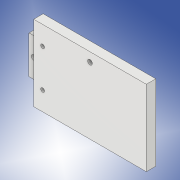
# Autodesk Inventor part: SP001
Saved by Autodesk Inventor 2017 SP1 (Build 210196100, 196)
## iProperties
Created: 2017-08-09
Part Number: SP001
Material: ABS Plastic
Document SubType Name: Modeling
Designer: Zach
Density: 1.06 g/cm^3
Appearance: CR White
Author: Zach
Autodesk Inventor part; units mm, degrees
ref_plane "YZ Plane" through (0, 0, 0) normal (1, 0, 0) x (0, 1, 0)
ref_plane "XZ Plane" through (0, 0, 0) normal (0, 1, 0) x (-1, 0, 0)
ref_plane "XY Plane" through (0, 0, 0) normal (0, 0, 1) x (1, 0, 0)
sketch "Sketch1" plane through (0, 0, 0) normal (0, 0, 1) x (1, 0, 0)
  line L0 (0, 0) -> (119, 0)
  line L1 (119, 0) -> (119, 80)
  line L2 (119, 80) -> (0, 80)
  line L3 (0, 80) -> (0, 0)
  dimension "d0" = 119
  dimension "d1" = 80
  constraints: 8 end point, 2 parallel, 1 horizontal, 1 perpendicular
  measures "d0" distance of L2.end L1.end
  measures "d1" distance of L1.end L0.end
extrude "Extrusion1" add sketch "Sketch1" along normal blind 10
sketch "Sketch2" plane through (0, 0, 10) normal (0, 0, 1) x (1, 0, 0)
  line L0 (-10, 60) -> (0, 60)
  line L1 (0, 60) -> (0, 20)
  line L2 (0, 20) -> (-10, 20)
  line L3 (-10, 20) -> (-10, 60)
  line L4 (0, 80) -> (0, 0) projected
  circle A0 centre (-5, 40) radius 2.5
  point P0 (0, 40)
  point P1 (0, 40)
  point P2 (0, 40)
  point P3 (0, 40)
  point P4 (-5, 60)
  dimension "d4" = 10
  dimension "d5" = 40
  dimension "d6" = 5
  constraints: 8 end point, 6 midpoint, 2 parallel, 1 centre point, 1 coincident, 1 horizontal, 1 horizontal alignment, 1 perpendicular, 1 vertical alignment
  measures "d4" distance of L1.end L2.end
  measures "d5" distance of L0.end L1.end
  measures "d6" diameter of A0
extrude "Extrusion2" add sketch "Sketch2" against normal blind 10
sketch "Sketch3" plane through (0, 0, 10) normal (0, 0, 1) x (1, 0, 0)
  circle A0 centre (9.5, 60) radius 2
  line L0 (0, 80) -> (0, 60) projected
  line L1 (119, 80) -> (0, 80) projected
  circle A1 centre (9.5, 20) radius 2
  point P0 (0, 0)
  dimension "d12" = 4
  dimension "d13" = 9.5
  dimension "d14" = 20
  dimension "d15" = 4
  dimension "d16" = 40
  constraints: 2 centre point, 1 vertical alignment
  measures "d12" diameter of A0
  measures "d13" distance from line of L0 A0.centre
  measures "d14" distance from line of L1 A0.centre
  measures "d15" diameter of A1
  measures "d16" distance of A1.centre A0.centre
extrude "Extrusion3" cut sketch "Sketch3" against normal through all
sketch "Sketch4" plane through (0, 0, 10) normal (0, 0, 1) x (1, 0, 0)
  line L0 (0, 80) -> (0, 60) projected
  line L1 (0, 20) -> (-10, 20) projected
  line L2 (0, 60) -> (-10, 60)
  line L3 (-10, 60) -> (-10, 20)
  line L4 (-10, 20) -> (0, 20)
  line L5 (0, 20) -> (0, 60)
  point P0 (0, 0)
  constraints: 8 end point, 2 parallel, 1 horizontal, 1 perpendicular
extrude "Extrusion4" cut sketch "Sketch4" against normal blind 5
sketch "Sketch5" plane through (0, 0, 10) normal (0, 0, 1) x (1, 0, 0)
  circle A0 centre (59.5, 70.5) radius 2.5
  line L0 (119, 80) -> (0, 80) projected
  point P0 (0, 0)
  point P1 (59.5, 80)
  dimension "d21" = 5
  dimension "d22" = 9.5
  constraints: 1 centre point, 1 midpoint, 1 vertical alignment
  measures "d21" diameter of A0
  measures "d22" distance from line of A0.centre L0
extrude "Extrusion5" cut sketch "Sketch5" against normal through all
body "Solid1"
